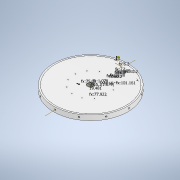
# Autodesk Inventor part: RotorBody
Saved by Autodesk Inventor 2022.2 (Build 262287000, 287)
## iProperties
Created: 2022-07-28
Part Number: RotorBody
Material: ABS Plastic
Document SubType Name: Modeling
Designer: ABL
Density: 1.06 g/cm^3
Appearance: Smooth - White
Author: ABL
Autodesk Inventor part; units mm, degrees
note: some values were not read from the file. Chosen so that the rebuilt part matches the saved one: direction of "halbachMagnet_removalHole".
ref_plane "Work Plane5" through (-27.2565, 0, -101.7227) normal (-0.258819, 0, -0.9659258) x (0, -1, 0)
sketch "Sketch2" plane through (0, 0, 0) normal (0, 1, 0) x (-1, 0, 0)
  circle A0 centre (0, 0) radius 101.1611
  circle A1 centre (0, 0) radius 4.2
  dimension "d4" = 202.3223
  dimension "d101" = 8.4
  constraints: 2 centre point, 2 coincident
  measures "d4" diameter of A0
  measures "d101" diameter of A1
extrude "Extrusion1" add sketch "Sketch2" along normal blind 14.1
ref_plane "Work Plane4" through (-26.1824, 0, -97.7141) normal (-0.258819, 0, -0.9659258) x (0, -1, 0)
sketch "Sketch13" plane through (-27.2565, 0, -101.7227) normal (-0.258819, 0, -0.9659258) x (0, -1, 0)
  line L0 (-14.1, 101.1611) -> (-14.1, -101.1611) construction
  line L1 (0, 0) -> (-14.1, 0) construction
  line L2 (0, 0.05) -> (-14.1, 0.05)
  line L3 (-14.1, 0.05) -> (-14.1, -0.05)
  line L4 (-14.1, -0.05) -> (0, -0.05)
  line L5 (0, -0.05) -> (0, 0.05)
  line L6 (0, 0.05) -> (-14.1, -0.05) construction
  line L7 (-14.1, 0.05) -> (0, -0.05) construction
  point P0 (-7.05, 0)
  dimension "d136" = 0.1
  dimension "d139" = 7.05
  dimension "d140" = 2.05
  dimension "d141" = 4.2
  dimension "d142" = 3.8
  dimension "d146" = 4.1
  dimension "d147" = 4.3
  dimension "d153" = 4.2
  constraints: 8 end point, 2 parallel, 1 horizontal, 1 perpendicular
  measures "d153" distance of L2.end L3.end
sketch "Sketch10" plane through (0, 0, 0) normal (0, -1, 0) x (1, 0, 0)
  line L0 (0, 0) -> (-27.2565, -101.7227)
  line L1 (0, 0) -> (105.3111, 0) construction
  arc A0 (-27.2565, -101.7227) -> (30.0421, -100.9352) centre (0, 0) ccw
  line L2 (0, 0) -> (30.0421, -100.9352)
  line L3 (0, 0) -> (-27.2565, -101.7227) construction
  dimension "d96" = 105.3111
  dimension "d97" = 105
  dimension "d98" = 31.575
  constraints: 8 end point, 2 point on circle, 1 centre point, 1 coincident, 1 equal length, 1 horizontal
  measures "d96" distance of L0.start L0.end
  measures "d97" angle of L0 L1
  measures "d98" angle of L3 L2
sketch "Sketch8" plane through (0, 0, 0) normal (0, 1, 0) x (-1, 0, 0)
  circle A0 centre (0, 0) radius 105.3111
  circle A1 centre (0, 0) radius 101.2111
  dimension "d81" = 210.6223
  dimension "d82" = 202.4223
  constraints: 2 centre point, 2 coincident
  measures "d81" diameter of A0
  measures "d82" diameter of A1
extrude "Extrusion2" add sketch "Sketch8" along normal blind 14.1 separate body
sketch "Sketch1" plane through (0, 0, 0) normal (0, 1, 0) x (-1, 0, 0)
  circle A0 centre (0, 0) radius 38.9611 construction
  arc A1 (-26.1824, -97.7141) -> (26.1824, -97.7141) centre (0, 0) ccw
  line L0 (0, 0) -> (26.1824, -97.7141)
  line L1 (0, 0) -> (101.1611, 0) construction
  line L2 (0, 0) -> (-26.1824, -97.7141)
  line L3 (26.1824, -97.7141) -> (10.0839, -37.6336)
  line L4 (-26.1824, -97.7141) -> (-10.0839, -37.6336)
  line L5 (-9.1685, -38.2045) -> (0.974, -39.2858)
  line L6 (0.974, -39.2858) -> (-5.4077, -99.1465)
  line L7 (-5.4077, -99.1465) -> (-15.5502, -98.0652)
  line L8 (-15.5502, -98.0652) -> (-9.1685, -38.2045)
  line L9 (0, 0) -> (0, -101.1611) construction
  line L10 (9.0751, -38.0161) -> (2.9494, -38.9728)
  line L11 (2.9494, -38.9728) -> (12.2391, -98.4517)
  line L12 (12.2391, -98.4517) -> (18.3649, -97.495)
  line L13 (18.3649, -97.495) -> (9.0751, -38.0161)
  line L14 (-4.0988, -38.7449) -> (0, 0) construction
  circle A2 centre (-2.0494, -19.3725) radius 2.6
  circle A3 centre (0, 0) radius 101.1611 construction
  line L15 (5.5465, -87.1678) -> (0.7497, -87.3409)
  line L16 (0.7497, -87.3409) -> (0.8218, -89.3396)
  line L17 (0.8218, -89.3396) -> (5.6187, -89.1665)
  line L18 (5.6187, -89.1665) -> (5.5465, -87.1678)
  line L19 (0, 0) -> (3.1481, -87.2544) construction
  line L20 (0.7497, -87.3409) -> (-4.0941, -86.8245) construction
  line L21 (5.5465, -87.1678) -> (10.3594, -86.4161) construction
  line L22 (3.2202, -89.2531) -> (3.6475, -101.0954) construction
  line L23 (-4.0988, -38.7449) -> (-5.1508, -48.6894) construction
  point P0 (6.0123, -38.4944)
  dimension "d0" = 77.9223
  dimension "d1" = 101.1611
  dimension "d2" = 75
  dimension "d3" = 30
  dimension "d7" = 10.2
  dimension "d8" = 60.2
  dimension "d9" = 6.2
  dimension "d10" = 60.2
  dimension "d11" = 2
  dimension "d15" = 1.0788
  dimension "d16" = 1.0788
  dimension "d17" = 5.2
  dimension "d66" = 4.8
  dimension "d67" = 2
  dimension "d79" = 90
  dimension "d80" = 11.85
  dimension "d108" = 19.4806
  dimension "d122" = 10
  constraints: 48 end point, 7 perpendicular, 7 point on circle, 4 midpoint, 4 parallel, 4 point on line, 3 centre point, 3 coincident, 2 collinear, 2 equal length, 2 tangent, 1 horizontal
  measures "d0" diameter of A0
  measures "d1" radius of A1
  measures "d2" angle of L0 L1
  measures "d3" angle of L2 L0
  measures "d7" distance of L6.end L7.end
  measures "d8" distance of L5.end L6.end
  measures "d9" distance of L12.end L11.end
  measures "d10" distance of L11.end L10.end
  measures "d11" distance of L10.end L5.end
  measures "d15" distance of L5.start L4.end
  measures "d16" distance of L3.end L10.start
  measures "d17" diameter of A2
  measures "d66" distance of L15.start L15.end
  measures "d67" distance of L15.end L16.end
  measures "d79" angle of L19 L15
  measures "d80" distance of L22.start L22.end
  measures "d108" distance of A0.centre A2.centre
  measures "d122" distance of L14.start L23.end
extrude "driveMagnet_slot" cut sketch "Sketch1" along normal blind 10.1 contours L5 L6 L7 L8 bodies 1
extrude "halbachMagnet_slot" cut sketch "Sketch1" along normal blind 12.1 contours L13 L12 L11 L10 bodies 1
sketch "Sketch4" plane through (-12.2391, 0, -98.4517) normal (0.1543146, 0, 0.9880218) x (0.9880218, 0, -0.1543146)
  line L0 (0, 0) -> (0, 12.1) projected
  line L1 (0, 2) -> (-6.2, 2)
  line L2 (-6.2, 2) -> (-6.2, 12.2)
  line L3 (-6.2, 12.2) -> (0, 12.2)
  line L4 (0, 12.2) -> (0, 2)
  line L5 (0, 0) -> (-6.2, 0) projected
  point P0 (-3.1, 0)
  point P1 (0, 12.1)
  dimension "d31" = 6.2
  dimension "halbachMagnet_slotHeight" = 10.2
  dimension "d33" = 2
  constraints: 8 end point, 2 parallel, 1 horizontal, 1 perpendicular, 1 point on line
  measures "d31" distance of L2.end L3.end
  measures "halbachMagnet_slotHeight" distance of L1.end L2.end
  measures "d33" distance between parallel lines of L5 L1
extrude "halbachMagnet_opening" cut sketch "Sketch4" against normal through all bodies 1
extrude "halbachMagnet_roof" add sketch "Sketch1" along normal blind 2 contours L13 L12 L11 L10 bodies 1
extrude "sensorMagnet_slot" cut sketch "Sketch1" along normal blind 2.7667 contours A2 bodies 1
extrude "rotorBandSquareNut_slot" cut sketch "Sketch1" along normal blind 9.2 contours L18 L17 L16 L15 bodies 1
pattern_circular "Circular Pattern1" count 12 over 360 about axis through (0, -10, 0) along (0, 1, 0) of "driveMagnet_slot", "halbachMagnet_slot", "sensorMagnet_slot", "halbachMagnet_opening", "halbachMagnet_roof", "rotorBandSquareNut_slot" bodies 1
sketch "Sketch7" plane through (-5.5465, 0, -87.1678) normal (-0.0360561, 0, -0.9993498) x (-0.9993498, 0, 0.0360561)
  line L0 (0, 9.2) -> (-4.8, 9.2) projected
  line L1 (-2.4, 9.2) -> (-2.4, 7.1) construction
  point P0 (-2.4, 0)
  dimension "d71" = 2.1
  constraints: 2 end point, 1 coincident, 1 midpoint, 1 vertical
  measures "d71" distance of L1.start L1.end
ref_plane "Work Plane2" through (-3.7971, 0, -105.2427) normal (0.0360561, 0, 0.9993498) x (0, 1, 0)
ref_plane "Work Plane1" through (-5.5465, 4.6, -87.1678) normal (0.0360561, 0, 0.9993498) x (0, 1, 0)
sketch "Sketch9" plane through (-3.7971, 0, -105.2427) normal (0.0360561, 0, 0.9993498) x (0, 1, 0)
  line L0 (0, 0) -> (7.05, 0) construction
  dimension "d85" = 7.05
  constraints: 2 coincident, 2 end point, 1 horizontal
  measures "d85" distance of L0.start L0.end
hole "rotorBandBolt_hole" at (-3.7971, 7.05, -105.2427) direction (0.0360561, 0, 0.9993498) diameter 2.4 depth 24 counterbore diameter 4.08 counterbore depth 2.1 bodies 2 1
pattern_circular "BoltHoles" count 12 over 360 about axis through (0, -10, 0) along (0, 1, 0) of "rotorBandBolt_hole" bodies 1 2
sketch "Sketch11" plane through (0, 0, 0) normal (0, -1, 0) x (1, 0, 0)
  circle A0 centre (0, 0) radius 9
  circle A1 centre (0, 0) radius 8
  dimension "d102" = 18
  dimension "d105" = 16
  constraints: 2 centre point, 2 coincident
  measures "d102" diameter of A0
  measures "d105" diameter of A1
extrude "flangeBearing_flangeInset" cut sketch "Sketch11" against normal blind 1 bodies 1
extrude "flangeBearing_bodyInset" cut sketch "Sketch11" against normal blind 5 contours A1 bodies 1
ref_plane "Work Plane3" through (0, 7.05, 0) normal (0, -1, 0) x (1, 0, 0)
mirror "flangeBearing_mirror" about plane through (0, 7.05, 0) normal (0, -1, 0) of "flangeBearing_flangeInset", "flangeBearing_bodyInset" bodies 1
hole "halbachMagnet_removalHole" at (-6.0123, 0, -38.4944) direction (0, 1, 0) diameter 2 depth 12.1 bodies 1
sketch "Sketch12" plane through (-9.0751, 2, -38.0161) normal (-0.1543146, 0, -0.9880218) x (-0.9880218, 0, 0.1543146)
  line L0 (-6.2, 0) -> (0, 0) projected
  line L1 (-3.1, 0) -> (-3.1, -2) construction
  line L2 (-3.1, -2) -> (-4.1, -2)
  line L3 (-4.1, -2) -> (-4.1, 0)
  line L4 (-4.1, 0) -> (-3.1, 0)
  line L5 (-3.1, -2) -> (-2.1, -2)
  line L6 (-2.1, -2) -> (-2.1, 0)
  line L7 (-2.1, 0) -> (-3.1, 0)
  point P0 (-2.1, 0)
  point P1 (-4.1, 0)
  dimension "d116" = 1
  constraints: 14 end point, 2 parallel, 2 symmetric about line, 1 midpoint, 1 perpendicular, 1 vertical
  measures "d116" distance of L1.end L2.end
extrude "halbachMagnet_removalChannel" cut sketch "Sketch12" along normal blind 10 bodies 1
hole "driveMagnet_removalHole" at (5.1508, 0, -48.6894) direction (0, 1, 0) diameter 2 depth 14.1 bodies 1
pattern_circular "Circular Pattern3" count 12 over 360 about axis through (0, -10, 0) along (0, 1, 0) of "halbachMagnet_removalHole", "halbachMagnet_removalChannel", "driveMagnet_removalHole" bodies 1
equation "\"d4\" = 2 * rotorRadius"
equation "\"d5\" = rotorThickness"
equation "\"d0\" = 2 * driveMagnet_centerSpacingRadius"
equation "\"d1\" = rotorRadius"
equation "\"d7\" = driveMagnet_width + 2 * gap"
equation "\"d8\" = driveMagnet_length + 2 * gap"
equation "\"d10\" = halbachMagnet_length + 2 * gap"
equation "\"d11\" = wallgap"
equation "\"d16\" = d15"
equation "\"d17\" = sensorMagnet_diameter + 2 * gap"
equation "\"d20\" = gap + halbachMagnet_width + wallgap"
equation "\"d33\" = wallgap"
equation "\"d36\" = wallgap"
equation "\"d22\" = sensorMagnet_height + gap"
equation "\"d68\" = 0.5 * rotorBandSquareNut_sideLength + 0.5 * halbachMagnet_slotHeight + wallgap + gap"
equation "\"d71\" = 0.5 * rotorBandSquareNut_sideLength + gap"
equation "\"gap\" = 0.1"
equation "\"airgap\" = 0.4"
equation "\"driveMagnet_height\" = 5"
equation "\"halbachMagnet_width\" = 10"
equation "\"halbachMagnet_height\" = 3"
equation "\"sensorMagnet_diameter\" = 5"
equation "\"sensorMagnet_height\" = 2.66667"
equation "\"wallgap\" = 2"
equation "\"driveMagnet_centerSpacingRadius\" = 38.96113"
equation "\"rotorThickness\" = 14.1"
equation "\"shaftDiameter\" = 8"
equation "\"flangeBearing_outerDiameter\" = 16"
equation "\"flangeBearing_innerDiameter\" = shaftDiameter"
equation "\"flangeBearing_height\" = 5"
equation "\"flangeBearing_flangeHeight\" = 1"
equation "\"flangeBearing_flangeDiameter\" = 18"
equation "\"statorThickness\" = 16"
equation "\"rotor_mountingLipHeight\" = 8"
equation "\"rotorRadius\" = 101.16113"
equation "\"rotorBandSquareNut_sideLength\" = 4"
equation "\"rotorBandHexNut_height\" = 1.2"
equation "\"rotorBandHexNut_sideToSide\" = 4"
equation "\"rotorBandSquareNut_height\" = 1.2"
equation "\"rotorBandBolt_headHeight\" = 2"
equation "\"rotorBandBolt_headDiameter\" = 3.98"
equation "\"rotorBandBolt_diameter\" = 2"
equation "\"rotorBandThickness\" = 4.1"
equation "\"flangeCoupling_collarOuterDiameter\" = 16"
equation "\"flangeCoupling_flangeHoleEdgeToEdge\" = 2.05"
equation "\"flangeCoupling_innerDiameter\" = 8"
equation "\"flangeCoupling_flangeHoleDiameter\" = 3.9"
equation "\"flangeCoupling_flangeHeight\" = 3.1"
equation "\"flangeCoupling_flangeDiameter\" = 32"
equation "\"flangeCoupling_height\" = 13.1"
equation "\"flangeCoupling_mountHoleDiameter\" = 3.9"
equation "\"flangeCoupling_mountHoleEdgeToEdge\" = 2.05"
equation "\"statorRadius\" = 99.16113"
equation "\"coilThickness\" = 12"
equation "\"statorMountBolt_diameter\" = 4"
equation "\"statorMountBolt_headDiameter\" = 7"
equation "\"statorMountBolt_headHeight\" = 4"
equation "\"statorMountBolt_shaftLength\" = 17.1"
equation "\"statorMountHexNut_height\" = 4"
equation "\"statorMountHexNut_sideToSide\" = 8"
equation "\"sensorMagnet_ringRadius\" = 23.48057"
equation "\"coil_percentCoverage\" = 0.6"
equation "\"statorSpokeDegrees\" = 4deg"
equation "\"coil_bulge\" = 3"
equation "\"statorCoilBolt_shaftLength\" = 12"
equation "\"statorCoilHexNut_height\" = 1.2"
equation "\"statorCoilBolt_headHeight\" = 2"
equation "\"statorCoilBolt_diameter\" = 2"
equation "\"statorCoilBolt_headDiameter\" = 3.98"
equation "\"statorCoilHexNut_sideToSide\" = 4"
equation "\"driveMagnet_width\" = 10"
equation "\"driveMagnet_length\" = 60"
equation "\"halbachMagnet_length\" = 60"
